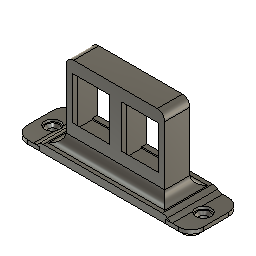
keystone (Autodesk Fusion 360 design; units mm, degrees)
Autodesk Fusion 360 part; units mm, degrees
sketch "Sketch1" plane through (0, 0, 0) normal (0, 0, 1) x (1, 0, 0)
  line L0 (0, 0) -> (-25, 0) construction
  line L1 (0, 0) -> (25, 0) construction
  line L2 (25, 0) -> (25, 10)
  line L3 (25, 0) -> (25, -10)
  line L4 (25, 10) -> (-25, 10)
  line L5 (-25, 10) -> (-25, 0)
  line L6 (-25, 0) -> (-25, -10)
  line L7 (-25, -10) -> (25, -10)
  line L8 (25, 10) -> (35, 10)
  line L9 (35, 10) -> (35, -10)
  line L10 (35, -10) -> (25, -10)
  line L11 (-25, 10) -> (-35, 10)
  line L12 (-35, 10) -> (-35, -10)
  line L13 (-35, -10) -> (-25, -10)
  line L14 (-35, -10) -> (-25, 10) construction
  line L15 (-35, 10) -> (-25, -10) construction
  line L16 (25, -10) -> (35, 10) construction
  line L17 (25, 10) -> (35, -10) construction
  circle A0 centre (-30, 0) radius 1.5
  circle A1 centre (-30, 0) radius 3
  circle A2 centre (30, 0) radius 1.5
  circle A3 centre (30, 0) radius 3
  dimension "d6" = 20
  dimension "d7" = 50
  dimension "d8" = 10
  dimension "d9" = 10
  dimension "d10" = 3
  dimension "d11" = 6
  dimension "d12" = 3
  dimension "d13" = 6
  constraint coincident L0.start L1.start
  constraint horizontal L0
  constraint parallel L0 L1
  constraint perpendicular L1 L2
  constraint perpendicular L1 L3
  constraint perpendicular L2 L4
  constraint perpendicular L0 L6
  constraint perpendicular L4 L5
  constraint perpendicular L6 L7
  constraint equal L2 L3
  constraint equal L0 L1
  constraint perpendicular L2 L8
  constraint perpendicular L8 L9
  constraint perpendicular L5 L11
  constraint perpendicular L11 L12
  constraint perpendicular L12 L13
  constraint midpoint L15 A0.centre
  constraint concentric A0 A1
  constraint midpoint L16 A2.centre
  constraint concentric A2 A3
  measures "d6" distance of L4 L7
  measures "d7" distance of L2.end L4.end
  measures "d8" distance of L2.end L8.end
  measures "d9" distance of L4.end L11.end
  measures "d10" diameter of A0
  measures "d11" diameter of A1
  measures "d12" diameter of A2
  measures "d13" diameter of A3
extrude "Extrude3" add sketch "Sketch1" along normal blind 5 contours L2 L3 L4 L5 L6 L7
extrude "Extrude2" add sketch "Sketch1" along normal blind 3.5 contours L2 L3 L4 L5 L6 L7 | L2 L3 L8 L9 L10 | L5 L6 L11 L12 L13
extrude "Extrude1" add sketch "Sketch1" along normal blind 2.5 contours L2 L3 L4 L5 L6 L7 | L2 L3 L8 L9 L10 | L5 L6 L11 L12 L13 | A1 | A3
fillet "Fillet1" radius 5 4 edges at (35, -10, 1.75) (35, 10, 1.75) (-35, 10, 1.75) (-35, -10, 1.75)
fillet "Fillet2" radius 3 2 edges at (25, 0, 3.5) (-25, 0, 3.5)
fillet "Fillet3" radius 3 2 edges at (25, 0, 5) (-25, 0, 5)
chamfer "Chamfer1" distance 1 angle 45 2 edges at (-31.3985, 0.5424, 2.5) (28.6015, 0.5424, 2.5)
sketch "Sketch2" plane through (0, 0, 5) normal (0, 0, 1) x (-1, 0, 0)
  line L0 (23.6294, -10) -> (23.6294, 10)
  line L1 (23.6294, 10) -> (-23.6294, 10)
  line L2 (-23.6294, 10) -> (-23.6294, -10)
  line L3 (-23.6294, -10) -> (23.6294, -10)
  line L4 (19.6294, -5) -> (-19.6294, -5)
  line L5 (-19.6294, -5) -> (-19.6294, 5)
  line L6 (-19.6294, 5) -> (19.6294, 5)
  line L7 (19.6294, 5) -> (19.6294, -5)
  line L8 (-25, -10) -> (25, -10)
  line L9 (25, 10) -> (-25, 10)
  dimension "d24" = 4
  dimension "d25" = 4
  dimension "d26" = 5
  dimension "d27" = 5
  constraint perpendicular L0 L4
  constraint perpendicular L4 L5
  constraint perpendicular L5 L6
  constraint perpendicular L4 L7
  measures "d24" distance of L0 L7
  measures "d25" distance of L2 L5
  measures "d26" distance of L4 L8
  measures "d27" distance of L6 L9
extrude "Extrude4" add sketch "Sketch2" along normal blind 30 contours L4 L5 L6 L7
fillet "Fillet4" radius 3.5 4 edges at (19.6294, 0, 5) (-19.6294, 0, 5) (0, 5, 5) (0, -5, 5)
fillet "Fillet5" radius 3 2 edges at (-19.6294, 0, 35) (19.6294, 0, 35)
sketch "Sketch3" plane through (0, 5, 0) normal (0, 1, 0) x (-1, 0, 0)
  line L0 (-19.6294, 8.5) -> (19.6294, 8.5)
  line L1 (19.6294, 8.5) -> (19.6294, 32)
  line L2 (16.6294, 35) -> (-16.6294, 35)
  line L3 (-19.6294, 32) -> (-19.6294, 8.5)
  line L4 (0, 35) -> (0, 0) construction
  line L5 (-17.1147, 30.25) -> (-2.5147, 30.25)
  line L6 (-2.5147, 30.25) -> (-2.5147, 13.25)
  line L7 (-2.5147, 13.25) -> (-17.1147, 13.25)
  line L8 (-17.1147, 13.25) -> (-17.1147, 30.25)
  line L9 (2.5147, 30.25) -> (17.1147, 30.25)
  line L10 (17.1147, 30.25) -> (17.1147, 13.25)
  line L11 (17.1147, 13.25) -> (2.5147, 13.25)
  line L12 (2.5147, 13.25) -> (2.5147, 30.25)
  line L13 (-2.5147, 30.25) -> (0, 30.25) construction
  line L14 (-17.1147, 30.25) -> (-19.6294, 30.25) construction
  line L15 (-2.5147, 30.25) -> (-2.5147, 35) construction
  line L16 (-17.1147, 13.25) -> (-17.1147, 8.5) construction
  line L17 (2.5147, 30.25) -> (2.5147, 35) construction
  line L18 (17.1147, 13.25) -> (17.1147, 8.5) construction
  line L19 (0, 30.25) -> (2.5147, 30.25) construction
  line L20 (17.1147, 13.25) -> (19.6294, 13.25) construction
  arc A0 (-16.6294, 35) -> (-19.6294, 32) centre (-16.6294, 32) ccw
  arc A1 (19.6294, 32) -> (16.6294, 35) centre (16.6294, 32) ccw
  dimension "d31" = 14.6
  dimension "d32" = 17
  constraint midpoint L2 L4.start
  constraint coincident L4.end origin
  constraint horizontal L5
  constraint vertical L6
  constraint horizontal L7
  constraint vertical L8
  constraint horizontal L9
  constraint vertical L10
  constraint horizontal L11
  constraint vertical L12
  constraint coincident L4 L13.end
  constraint perpendicular L4 L13
  constraint coincident L3 L14.end
  constraint perpendicular L3 L14
  constraint equal L13 L14
  constraint coincident L2 L15.end
  constraint perpendicular L2 L15
  constraint coincident L0 L16.end
  constraint perpendicular L0 L16
  constraint equal L15 L16
  constraint coincident L2 L17.end
  constraint perpendicular L2 L17
  constraint coincident L0 L18.end
  constraint perpendicular L0 L18
  constraint equal L17 L18
  constraint coincident L1 L20.end
  constraint perpendicular L1 L20
  constraint equal L19 L20
  constraint equal L5 L9
  constraint equal L6 L12
  measures "d31" distance of L5.start L5.end
  measures "d32" distance of L5.start L7.end
extrude "Extrude5" cut sketch "Sketch3" against normal blind 10 contours L5 L6 L7 L8 | L9 L10 L11 L12
sketch "Sketch4" plane through (0, 5, 0) normal (0, 1, 0) x (-1, 0, 0)
  line L0 (-2.5147, 30.25) -> (-2.5147, 13.25)
  line L1 (-2.5147, 13.25) -> (-17.1147, 13.25)
  line L2 (-17.1147, 13.25) -> (-17.1147, 30.25)
  line L3 (-17.1147, 30.25) -> (-2.5147, 30.25)
  line L4 (17.1147, 30.25) -> (17.1147, 13.25)
  line L5 (17.1147, 13.25) -> (2.5147, 13.25)
  line L6 (2.5147, 13.25) -> (2.5147, 30.25)
  line L7 (2.5147, 30.25) -> (17.1147, 30.25)
  arc A0 (-16.6294, 35) -> (-19.6294, 32) centre (-16.6294, 32) ccw
  line L8 (-19.6294, 32) -> (-19.6294, 8.5)
  line L9 (-19.6294, 8.5) -> (19.6294, 8.5)
  line L10 (19.6294, 8.5) -> (19.6294, 32)
  arc A1 (19.6294, 32) -> (16.6294, 35) centre (16.6294, 32) ccw
  line L11 (16.6294, 35) -> (-16.6294, 35)
  line L12 (-2.5147, 30.25) -> (-2.5147, 13.25)
  line L13 (-17.1147, 30.25) -> (-2.5147, 30.25)
  line L14 (-17.1147, 13.25) -> (-17.1147, 30.25)
  line L15 (-2.5147, 13.25) -> (-17.1147, 13.25)
  line L16 (17.1147, 30.25) -> (17.1147, 13.25)
  line L17 (17.1147, 13.25) -> (2.5147, 13.25)
  line L18 (2.5147, 13.25) -> (2.5147, 30.25)
  line L19 (2.5147, 30.25) -> (17.1147, 30.25)
  line L20 (-17.2147, 31.75) -> (-2.4147, 31.75)
  line L21 (-2.4147, 31.75) -> (-2.4147, 10.25)
  line L22 (-2.4147, 10.25) -> (-17.2147, 10.25)
  line L23 (-17.2147, 10.25) -> (-17.2147, 31.75)
  line L24 (2.4147, 31.75) -> (17.2147, 31.75)
  line L25 (17.2147, 31.75) -> (17.2147, 10.25)
  line L26 (17.2147, 10.25) -> (2.4147, 10.25)
  line L27 (2.4147, 10.25) -> (2.4147, 31.75)
  dimension "d38" = 3
  dimension "d39" = 0.1
  dimension "d40" = 0.1
  dimension "d41" = 1.5
  dimension "d42" = 0.1
  dimension "d43" = 0.1
  dimension "d44" = 3
  dimension "d45" = 1.5
  constraint horizontal L20
  constraint vertical L21
  constraint horizontal L22
  constraint vertical L23
  constraint horizontal L24
  constraint vertical L25
  constraint horizontal L26
  constraint vertical L27
  measures "d38" distance of L1 L22
  measures "d39" distance of L0 L21
  measures "d40" distance of L14 L23
  measures "d41" distance of L3 L20
  measures "d42" distance of L18 L27
  measures "d43" distance of L4 L25
  measures "d44" distance of L5 L26
  measures "d45" distance of L19 L24
extrude "Extrude6" cut sketch "Sketch4" against normal blind 8 contours L20 L21 L22 L23 | L24 L25 L26 L27
sketch "Sketch5" plane through (0, 0, 10.25) normal (0, 0, 1) x (-1, 0, 0)
  line L0 (-17.2147, -5) -> (-2.4147, -5)
  line L1 (-2.4147, -5) -> (-2.4147, 3)
  line L2 (-2.4147, 3) -> (-17.2147, 3)
  line L3 (-17.2147, 3) -> (-17.2147, -5)
  line L4 (-17.1147, 3) -> (-2.5147, 3)
  line L5 (-2.5147, 3) -> (-2.5147, 5)
  line L6 (-2.5147, 5) -> (-17.1147, 5)
  line L7 (-17.1147, 5) -> (-17.1147, 3)
  line L8 (2.4147, -5) -> (17.2147, -5)
  line L9 (17.2147, -5) -> (17.2147, 3)
  line L10 (17.2147, 3) -> (2.4147, 3)
  line L11 (2.4147, 3) -> (2.4147, -5)
  line L12 (2.5147, 3) -> (17.1147, 3)
  line L13 (17.1147, 3) -> (17.1147, 5)
  line L14 (17.1147, 5) -> (2.5147, 5)
  line L15 (2.5147, 5) -> (2.5147, 3)
  line L16 (2.4147, -3) -> (17.2147, -3)
  line L17 (-2.4147, -3) -> (-17.2147, -3)
  dimension "d49" = 8
  dimension "d50" = 8
  constraint coincident L11 L16.start
  constraint coincident L9 L16.end
  constraint perpendicular L9 L16
  constraint coincident L1 L17.start
  constraint coincident L3 L17.end
  constraint perpendicular L1 L17
  measures "d49" distance of L14 L16
  measures "d50" distance of L6 L17
extrude "Extrude7" add sketch "Sketch5" along normal blind 0.5 contours L0 L1 L3 L17 | L8 L9 L11 L16
sketch "Sketch6" plane through (0, 0, 31.75) normal (0, 0, -1) x (1, 0, 0)
  line L0 (2.4147, -5) -> (17.2147, -5)
  line L1 (17.2147, -5) -> (17.2147, 3)
  line L2 (17.2147, 3) -> (2.4147, 3)
  line L3 (2.4147, 3) -> (2.4147, -5)
  line L4 (-2.4147, -5) -> (-17.2147, -5)
  line L5 (-17.2147, -5) -> (-17.2147, -3)
  line L6 (-17.2147, -3) -> (-2.4147, -3)
  line L7 (-2.4147, -3) -> (-2.4147, -5)
  line L8 (2.4147, -3) -> (17.2147, -3)
  line L9 (17.2147, -3) -> (17.2147, -5)
  line L10 (17.2147, -5) -> (2.4147, -5)
  line L11 (2.4147, -5) -> (2.4147, -3)
extrude "Extrude8" add sketch "Sketch6" along normal blind 0.5 contours L0 L1 L3 L8 L9 L10 L11 | L4 L5 L6 L7
chamfer "Chamfer2" distance 2 angle 55 2 edges at (9.8147, -3, 13.25) (-9.8147, -3, 13.25) measured on face at (7.3814, -3.6667, 13.25) measured on face at (-12.2481, -3.6667, 13.25)
chamfer "Chamfer3" distance 2 angle 45 10 edges at (-35, 0, 0) (-33.5355, -8.5355, 0) (-27.5, -10, 0) (0, -10, 0) (27.5, -10, 0) (33.5355, -8.5355, 0) (35, 0, 0) (33.5355, 8.5355, 0) (0, 10, 0) (-33.5355, 8.5355, 0)
named bodies: "keystone mount"
